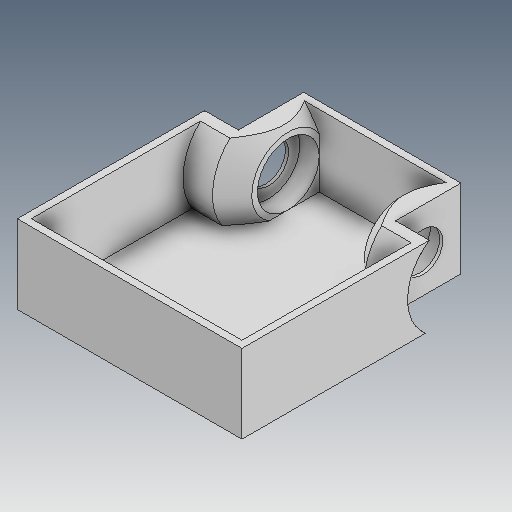
# Autodesk Inventor part: Base
Saved by Autodesk Inventor 2026.1 (Build 301233020, 233B)
## iProperties
Created: 2025-11-09
Part Number: Base
Material: Genérico
Document SubType Name: Modeling
Designer: Emmanuel Ribeiro
Density: 1 g/cm^3
Appearance: Padrão
Author: Emmanuel Ribeiro
Autodesk Inventor part; units mm, degrees
ref_plane "YZ Plane" through (0, 0, 0) normal (1, 0, 0) x (0, 1, 0)
ref_plane "XZ Plane" through (0, 0, 0) normal (0, 1, 0) x (-1, 0, 0)
sketch "Esboço1" plane through (0, 0, 0) normal (0, 1, 0) x (-1, 0, 0)
  line L0 (-50, 50) -> (50, 50)
  line L1 (50, 50) -> (50, -50)
  line L2 (50, -50) -> (-50, -50)
  line L3 (-50, -50) -> (-50, 50)
  line L4 (-50, 50) -> (50, -50) construction
  line L5 (50, 50) -> (-50, -50) construction
  point P0 (0, 0)
  dimension "d0" = 100
  dimension "d1" = 100
  constraints: 12 end point, 2 midpoint, 2 parallel, 1 horizontal, 1 perpendicular
  measures "d0" distance of L1.end L2.end
  measures "d1" distance of L0.end L1.end
extrude "Extrusão1" add sketch "Esboço1" along normal blind 28
sketch "Esboço3" plane through (0, 28, 0) normal (0, 1, 0) x (1, 0, 0)
  line L0 (50, 50) -> (-50, 50) projected
  line L1 (-40, 50) -> (40, 50)
  line L2 (-40, 50) -> (-40, -40)
  line L3 (-40, -40) -> (40, -40)
  line L4 (40, -40) -> (40, 50)
  point P0 (0, 0)
  point P1 (0, 50)
  dimension "d5" = 80
  dimension "d6" = 90
  constraints: 8 end point, 2 midpoint, 2 perpendicular, 1 point on line, 1 vertical
  measures "d5" distance of L1.start L1.end
  measures "d6" distance of L1.start L2.end
extrude "Extrusão2" cut sketch "Esboço3" against normal blind 28 keep common part
shell "Casca2" thickness 2.5 removed faces 1 at (-13.3333, 28, 10)
ref_plane "Plano de trabalho1" through (0, 28, 40) normal (1, 0, 0) x (0, 0, -1)
sketch "Esboço4" plane through (40, 28, 40) normal (1, 0, 0) x (0, 0, -1)
  circle A0 centre (76.5, -14.5) radius 17.5
  line L0 (90, -28) -> (90, 0) projected
  line L1 (0, -28) -> (90, -28) projected
  circle A1 centre (76.5, -14.5) radius 16.1
  circle A2 centre (76.5, -14.5) radius 11
  line L2 (87.5, -25.5) -> (87.5, 0) projected
  line L3 (2.5, -25.5) -> (87.5, -25.5) projected
  line L4 (90, 0) -> (66.702, 0)
  line L5 (90, 0) -> (90, -28) projected
  line L6 (90, -28) -> (87.6355, -28)
  point P0 (40, -28)
  point P1 (90, -25.6355)
  point P2 (90, -3.3645)
  point P3 (86.298, 0)
  dimension "d11" = 35
  dimension "d14" = 32.2
  dimension "d15" = 22
  constraints: 4 end point, 3 centre point, 2 coincident, 2 point on circle, 2 tangent, 1 horizontal, 1 point on line, 1 other
  measures "d11" diameter of A0
  measures "d14" diameter of A1
  measures "d15" diameter of A2
extrude "Extrusão3" cut sketch "Esboço4" against normal blind 12
sketch "Esboço5" plane through (28, 28, 40) normal (1, 0, 0) x (0, 0, -1)
  arc A0 (66.702, 0) -> (65.3645, -28) centre (76.5, -14.5) ccw projected
  arc A1 (65.3023, 2.0714) -> (63.7737, -29.9286) centre (76.5, -14.5) ccw
  line L0 (65.3645, -28) -> (61.7436, -28)
  line L1 (90, -28) -> (0, -28) projected
  line L2 (66.702, 0) -> (62.725, 0)
  point P0 (40, -28)
  dimension "d18" = 2.5
  constraints: 4 end point, 4 point on circle, 1 centre point, 1 parallel, 1 point on line
  measures "d18" radial gap between concentric circles of A0 A1
extrude "Extrusão4" add sketch "Esboço5" along normal up to surface (12 mm away)
sketch "Esboço6" plane through (28, 28, 40) normal (-1, 0, 0) x (0, 0, 1)
  arc A0 (-59.7967, -25.5) -> (-62.725, 0) centre (-76.5, -14.5) ccw projected
  line L0 (-66.702, 0) -> (-62.725, 0) projected
  line L1 (-87.5, -25.5) -> (-87.5, 0) projected
  line L2 (-87.5, -25.5) -> (-59.7967, -25.5)
  line L3 (-87.5, 0) -> (-66.702, 0)
  point P0 (-40, -28)
  constraints: 4 end point, 2 horizontal
extrude "Extrusão5" add sketch "Esboço6" along normal blind 8
sketch "Esboço7" plane through (20, 28, 40) normal (-1, 0, 0) x (0, 0, 1)
  arc A0 (-59.7967, -25.5) -> (-62.725, 0) centre (-76.5, -14.5) ccw projected
  circle A1 centre (-76.5, -14.5) radius 11
  point P0 (-40, -28)
  dimension "d23" = 22
  constraints: 1 centre point, 1 coincident
  measures "d23" diameter of A1
extrude "Extrusão6" cut sketch "Esboço7" against normal blind 6.9
chamfer "Chanfro1" distance 7 angle 45 1 edges at (20, 15.7817, -16.6306)
sketch "Esboço8" plane through (28, 28, 40) normal (1, 0, 0) x (0, 0, -1)
  arc A0 (66.702, 0) -> (65.3645, -28) centre (76.5, -14.5) ccw projected
  circle A1 centre (76.5, -14.5) radius 7
  point P0 (40, -28)
  dimension "d29" = 14
  constraints: 1 centre point, 1 coincident
  measures "d29" diameter of A1
extrude "Extrusão7" cut sketch "Esboço8" against normal blind 8
mirror "Espelhar1" about plane through (0, 28, 40) normal (1, 0, 0) of "Extrusão3", "Extrusão4", "Extrusão5", "Extrusão6", "Chanfro1", "Extrusão7"
